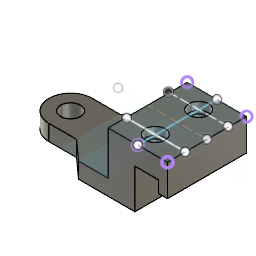
MARS_2 (Autodesk Fusion 360 design; units mm, degrees)
part number: 2026-05-31-13-57-16-867
Autodesk Fusion 360 part; units mm, degrees
sketch "Sketch1" plane through (0, 0, 0) normal (0, 0, 1) x (1, 0, 0)
  line L0 (112.5, -100) -> (-112.5, -100)
  line L1 (-112.5, -100) -> (-112.5, 100)
  line L2 (-112.5, 100) -> (112.5, 100)
  line L3 (112.5, 100) -> (112.5, -100)
  line L4 (112.5, -100) -> (-112.5, 100) construction
  line L5 (-112.5, -100) -> (112.5, 100) construction
  line L6 (0, 100) -> (0, -100) construction
  line L7 (-112.5, 0) -> (112.5, 0) construction
  dimension "d1" = 225
  dimension "d2" = 200
  constraint horizontal L0
  constraint perpendicular L0 L1
  constraint parallel L0 L2
  constraint parallel L1 L3
  constraint coincident L4 origin
  constraint coincident L5 origin
  constraint midpoint L2 L6.start
  constraint perpendicular L2 L6
  constraint midpoint L1 L7.start
  constraint midpoint L3 L7.end
  measures "d1" distance of L1.end L2.end
  measures "d2" distance of L0.end L1.end
extrude "Extrude1" add sketch "Sketch1" along normal blind 150
sketch "Sketch2" plane through (0, 100, 0) normal (0, 1, 0) x (-1, 0, 0)
  line L0 (-112.5, 0) -> (112.5, 0)
  line L1 (112.5, 0) -> (112.5, 150)
  line L2 (112.5, 150) -> (-112.5, 150)
  line L3 (-112.5, 150) -> (-112.5, 0)
  line L4 (112.5, 150) -> (37.5, 150)
  line L5 (37.5, 150) -> (37.5, 40)
  line L6 (37.5, 40) -> (112.5, 40)
  line L7 (112.5, 40) -> (112.5, 150)
  dimension "d5" = 75
  constraint horizontal L4
  constraint vertical L5
  constraint horizontal L6
  constraint vertical L7
  constraint coincident L1.end L2.start
  measures "d5" distance of L5.end L6.end
sketch "Sketch3" plane through (0, 100, 0) normal (0, 1, 0) x (-1, 0, 0)
extrude "Extrude2" cut sketch "Sketch2" against normal blind 540 contours L1 L2 L4 L5 L6 L7
sketch "Sketch4" plane through (0, 100, 0) normal (0, 1, 0) x (-1, 0, 0)
  line L0 (112.5, 40) -> (37.5, 40)
  line L1 (37.5, 40) -> (37.5, 150)
  line L2 (37.5, 150) -> (-112.5, 150)
  line L3 (-112.5, 150) -> (-112.5, 0)
  line L4 (-112.5, 0) -> (112.5, 0)
  line L5 (112.5, 0) -> (112.5, 40)
sketch "Sketch5" plane through (0, 0, 150) normal (0, 0, 1) x (-1, 0, 0)
  line L0 (37.5, -100) -> (37.5, 100)
  line L1 (37.5, 100) -> (-112.5, 100)
  line L2 (-112.5, 100) -> (-112.5, -100)
  line L3 (-112.5, -100) -> (37.5, -100)
sketch "Sketch6" plane through (0, 100, 0) normal (0, 1, 0) x (-1, 0, 0)
  line L0 (-112.5, 0) -> (-112.5, 70)
  line L1 (-112.5, 70) -> (-90, 70)
  line L2 (-90, 70) -> (-90, 100)
  line L3 (-90, 100) -> (-30, 100)
  line L4 (-30, 100) -> (-30, 0)
  line L5 (-30, 0) -> (-112.5, 0)
  line L6 (37.5, 150) -> (-112.5, 150)
  point P0 (37.5, 150)
  point P1 (37.5, 40)
  point P2 (-112.5, 0)
  dimension "d8" = 50
  dimension "d9" = 80
  dimension "d10" = 110
  dimension "d11" = 150
  constraint vertical L0
  constraint perpendicular L0 L1
  constraint perpendicular L1 L2
  constraint perpendicular L2 L3
  constraint perpendicular L3 L4
  constraint perpendicular L0 L5
  measures "d8" distance of L2.end L6
  measures "d9" distance of L0.end L6.end
  measures "d10" distance of P0 P1
  measures "d11" distance of L6.end P2
extrude "Extrude3" cut sketch "Sketch6" against normal blind 375
sketch "Sketch7" plane through (0, 0, 150) normal (0, 0, 1) x (-1, 0, 0)
  line L0 (-37.5, 100) -> (-37.5, -100) construction
  line L1 (-112.7809, 55) -> (35.5051, 55) construction
  line L2 (-110, -55) -> (40, -55) construction
  point P0 (-112.5, 100)
  point P1 (37.5, -100)
  dimension "d14" = 75
  dimension "d15" = 45
  dimension "d16" = 45
  constraint vertical L0
  constraint horizontal L1
  constraint horizontal L2
  measures "d14" distance of L0.start P0
  measures "d15" vertical distance of P0 L1.start
  measures "d16" vertical distance of L2.end P1
sketch "Sketch8" plane through (0, 0, 150) normal (0, 0, 1) x (-1, 0, 0)
  line L0 (-37.5, 100) -> (-37.5, -100)
  point P0 (-112.5, -100)
  dimension "d17" = 75
  constraint vertical L0
  measures "d17" distance of L0.end P0
sketch "Sketch9" plane through (0, 100, 0) normal (0, 1, 0) x (-1, 0, 0)
  point P0 (-112.7809, 150)
  point P1 (37.5, 150)
sketch "Sketch10" plane through (0, 0, 150) normal (0, 0, 1) x (-1, 0, 0)
  line L0 (-111.7438, 55) -> (36.0063, 55)
  line L1 (112.5, 0) -> (-112.3459, 0) construction
  line L2 (40, -55) -> (-112.822, -55) construction
  point P0 (-112.5, 100)
  point P1 (-37.5, 100)
  point P2 (-112.5, 100)
  point P3 (40, -55)
  point P4 (37.5, -100)
  dimension "d19" = 75
  dimension "d20" = 45
  dimension "d21" = 45
  constraint horizontal L0
  constraint horizontal L1
  constraint coincident P3 L2.start
  constraint horizontal L2
  measures "d19" distance of P0 P1
  measures "d20" vertical distance of L0.start P2
  measures "d21" vertical distance of P3 P4
sketch "Sketch11" plane through (0, 0, 150) normal (0, 0, 1) x (-1, 0, 0)
hole "Hole1" at (36.2725, -54.6667, 150) direction (0, 0, -1) diameter 30 depth 50 tip angle 180 counterbore diameter 50 counterbore depth 20
hole "Hole2" at (36.4807, 55.0076, 150) direction (0, 0, -1) diameter 30 depth 50 tip angle 180 counterbore diameter 50 counterbore depth 20
sketch "Sketch12" plane through (0, 0, 40) normal (0, 0, 1) x (-1, 0, 0)
  line L0 (112.5, 100) -> (37.5, 100)
  line L1 (37.5, 100) -> (37.5, -100)
  line L2 (37.5, -100) -> (112.5, -100)
  line L3 (112.5, -100) -> (112.5, 100)
sketch "Sketch13" plane through (0, 0, 40) normal (0, 0, 1) x (-1, 0, 0)
sketch "Sketch14" plane through (0, 0, 40) normal (0, 0, 1) x (-1, 0, 0)
sketch "Sketch15" plane through (0, 0, 40) normal (0, 0, 1) x (-1, 0, 0)
sketch "Sketch16" plane through (0, 0, 40) normal (0, 0, 1) x (-1, 0, 0)
  line L0 (112.5, -100) -> (112.5, 100)
  line L1 (112.5, 100) -> (162.5, 100)
  line L2 (162.5, 100) -> (162.5, -100)
  line L3 (162.5, -100) -> (112.5, -100)
  dimension "d40" = 50
  dimension "d41" = 200
  dimension "d42" = 50
  constraint vertical L0
  constraint perpendicular L0 L1
  constraint perpendicular L1 L2
  constraint perpendicular L2 L3
  measures "d40" distance of L0.end L1.end
  measures "d41" distance of L1.end L2.end
  measures "d42" distance of L2.end L0.start
extrude "Extrude4" add sketch "Sketch16" against normal blind 40
sketch "Sketch17" plane through (0, 0, 40) normal (0, 0, 1) x (-1, 0, 0)
  line L0 (112.5, 100) -> (37.5, 100)
  line L1 (37.5, 100) -> (37.5, -100)
  line L2 (37.5, -100) -> (112.5, -100)
  line L3 (112.5, -100) -> (162.5, -100)
  line L4 (162.5, -100) -> (162.5, 100)
  line L5 (162.5, 100) -> (112.5, 100)
sketch "Sketch18" plane through (0, 0, 40) normal (0, 0, 1) x (-1, 0, 0)
  line L0 (162.3989, 55) -> (162.5, 55)
  line L1 (162.5, -55) -> (162.485, -55)
  line L2 (162.5, -55) -> (162.5, -100)
  line L3 (162.5, -100) -> (112.5, -100)
  line L4 (162.5, -100) -> (112.5, -100)
  line L5 (112.5, -100) -> (162.5, -55)
  line L6 (112.5, 0) -> (-112.3459, 0)
  line L7 (162.5, 100) -> (112.5, 100)
  line L8 (112.5, 100) -> (162.5, 55)
  line L9 (162.5, 55) -> (162.5, 100)
  point P0 (162.5, -100)
  point P1 (162.5, 100)
  dimension "d45" = 45
  dimension "d46" = 45
  dimension "d47" = 50
  dimension "d48" = 50
  constraint horizontal L0
  constraint horizontal L1
  constraint coincident P0 L2.end
  constraint perpendicular L2 L3
  constraint perpendicular L2 L4
  constraint symmetric L1.start L6 L0.end
  constraint symmetric P0 L6 P1
  constraint symmetric L3.end L6 L7.end
  measures "d45" vertical distance of L1.start P0
  measures "d46" vertical distance of L0.start L7.start
  measures "d47" distance of P0 L3.end
  measures "d48" distance of P0 L3.end
extrude "Extrude5" cut sketch "Sketch18" against normal blind 40
sketch "Sketch19" plane through (0, 0, 40) normal (0, 0, 1) x (-1, 0, 0)
  line L0 (162.5, -55) -> (232.5, -55)
  line L1 (162.5, 55) -> (232.5, 55)
  line L2 (162.5, -55) -> (162.5, 55)
  circle A0 centre (232.5, 0) radius 25
  arc A1 (232.5, -55) -> (232.5, 55) centre (232.5, 0) ccw
  line L3 (162.5, -100) -> (162.5, 100)
  point P0 (37.5, 100)
  point P1 (37.5, -100)
  dimension "d51" = 70
  dimension "d52" = 70
  dimension "d53" = 45
  dimension "d54" = 45
  dimension "d55" = 50
  constraint horizontal L0
  constraint horizontal L1
  constraint perpendicular L1 L2
  constraint tangent L0 A1
  constraint coincident A0.centre A1.centre
  constraint coincident L0.start L3
  measures "d51" distance of L0.start L0.end
  measures "d52" distance of L1.start L1.end
  measures "d53" vertical distance of L1.start P0
  measures "d54" vertical distance of L0.start P1
  measures "d55" diameter of A0
extrude "Extrude6" add sketch "Sketch19" against normal blind 40
